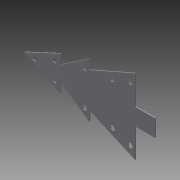
# Autodesk Inventor part: Arbol
Saved by Autodesk Inventor 2015 (Build 190159000, 159)
## iProperties
Created: 2016-11-22
Part Number: Arbol
Material: Generic
Document SubType Name: Modeling
Designer: Eduard
Density: 1 g/cm^3
Appearance: Default
Author: Eduard
Autodesk Inventor part; units mm, degrees
ref_plane "YZ Plane" through (0, 0, 0) normal (1, 0, 0) x (0, 1, 0)
ref_plane "XZ Plane" through (0, 0, 0) normal (0, 1, 0) x (-1, 0, 0)
ref_plane "XY Plane" through (0, 0, 0) normal (0, 0, 1) x (1, 0, 0)
sketch "Sketch1" plane through (0, 0, 0) normal (0, 1, 0) x (-1, 0, 0)
  line L0 (-128.7932, -21.9318) -> (-128.8163, -31.0141)
  line L1 (11.205, -31.37) -> (11.2067, -30.7124)
  line L2 (11.2067, -30.7124) -> (-27.3951, -12.7346)
  line L3 (-27.3951, -12.7346) -> (-27.3951, -23.154)
  line L4 (-27.3951, -23.154) -> (-58.7933, -1.6646)
  line L5 (-58.7933, -1.6646) -> (-58.7933, -12.2738)
  line L6 (-58.7933, -12.2738) -> (-107.4995, 9.0183)
  line L7 (-107.4995, 9.0183) -> (-107.4995, -21.9859)
  line L8 (-107.4995, -21.9859) -> (-128.7932, -21.9318)
  line L9 (-128.8163, -40.0964) -> (-128.8163, -31.0141)
  line L10 (11.205, -31.37) -> (-27.3968, -49.3478)
  line L11 (-27.3968, -49.3478) -> (-27.3968, -38.9284)
  line L12 (-27.3968, -38.9284) -> (-58.795, -60.4178)
  line L13 (-58.795, -60.4178) -> (-58.795, -49.8086)
  line L14 (-58.795, -49.8086) -> (-107.5012, -71.1006)
  line L15 (-107.5012, -71.1006) -> (-107.5012, -40.0964)
  line L16 (-107.5012, -40.0964) -> (-128.8163, -40.0964)
  circle A0 centre (0, -31.0141) radius 2.5
  circle A1 centre (-21.3305, -22.0944) radius 2.5
  circle A2 centre (-53.494, -12.7333) radius 2.5
  circle A3 centre (-102.2495, -1.636) radius 2.5
  circle A4 centre (-83.1694, -8.6081) radius 2.5
  circle A5 centre (-21.3772, -40.48) radius 2.5
  circle A6 centre (-53.5879, -49.6775) radius 2.5
  circle A7 centre (-102.3992, -60.5268) radius 2.5
  circle A8 centre (-83.2839, -53.6519) radius 2.5
  point P0 (0, 0)
  dimension "d2" = 5
  dimension "d3" = 5
  dimension "d4" = 5
  dimension "d5" = 5
  dimension "d6" = 5
  constraints: 34 end point, 9 centre point, 3 parallel, 1 perpendicular, 1 vertical
  measures "d2" diameter of A0
  measures "d3" diameter of A1
  measures "d4" diameter of A2
  measures "d5" diameter of A3
  measures "d6" diameter of A4
extrude "Extrusion1" add sketch "Sketch1" along normal blind 1
body "Solid1"
